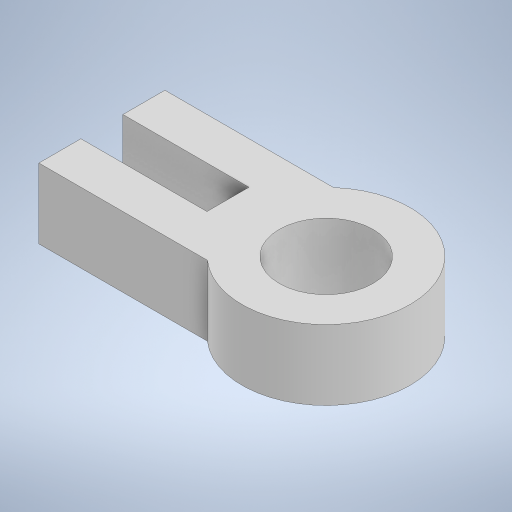
# Autodesk Inventor part: link_end_fixation
Saved by Autodesk Inventor 2024 (Build 280153000, 153)
## iProperties
Created: 2024-02-23
Part Number: link_end_fixation
Material: Generic
Document SubType Name: Modeling
Designer: clbri
Density: 1 g/cm^3
Appearance: Default
Author: clbri
Autodesk Inventor part; units mm, degrees
ref_plane "YZ Plane" through (0, 0, 0) normal (1, 0, 0) x (0, 1, 0)
ref_plane "XZ Plane" through (0, 0, 0) normal (0, 1, 0) x (-1, 0, 0)
ref_plane "XY Plane" through (0, 0, 0) normal (0, 0, 1) x (1, 0, 0)
sketch "Sketch1" plane through (0, 0, 0) normal (0, 0, 1) x (1, 0, 0)
  line L0 (0, 0) -> (13, 0)
  line L1 (13, 0) -> (13, 5)
  line L2 (13, 5) -> (0, 5)
  line L3 (0, 5) -> (0, 0)
  dimension "d0" = 13
  dimension "d1" = 5
  constraints: 8 end point, 2 parallel, 1 horizontal, 1 perpendicular
  measures "d0" distance of L2.end L1.end
  measures "d1" distance of L1.end L0.end
extrude "Extrusion1" add sketch "Sketch1" along normal blind 9
sketch "Sketch2" plane through (0, 5, 0) normal (0, 1, 0) x (1, 0, 0)
  line L0 (0, 0) -> (0, -9) projected
  line L1 (0, -6) -> (9, -6)
  line L2 (9, -6) -> (9, -3)
  line L3 (9, -3) -> (0, -3)
  line L4 (0, -3) -> (0, -6)
  line L5 (13, 0) -> (0, 0) projected
  point P0 (6.5, 0)
  point P1 (0, -3)
  dimension "d4" = 9
  dimension "d5" = 3
  dimension "d6" = 3
  constraints: 8 end point, 2 parallel, 1 horizontal, 1 midpoint, 1 perpendicular, 1 point on line
  measures "d4" distance of L3.end L2.end
  measures "d5" distance of L2.end L1.end
  measures "d6" distance from line of point (6.5, 0) L3
extrude "Extrusion2" cut sketch "Sketch2" against normal through all
sketch "Sketch3" plane through (0, 5, 0) normal (0, 1, 0) x (1, 0, 0)
  circle A0 centre (16, -4.5) radius 3.25
  circle A1 centre (16, -4.5) radius 6
  line L0 (9, -3) -> (9, -6) projected
  line L1 (13, 0) -> (0, 0) projected
  dimension "d9" = 6.5
  dimension "d10" = 12
  dimension "d11" = 7
  dimension "d12" = 4.5
  constraints: 2 centre point, 1 coincident
  measures "d9" diameter of A0
  measures "d10" diameter of A1
  measures "d11" distance from line of L0 A1.centre
  measures "d12" distance from line of L1 A0.centre
extrude "Extrusion3" add sketch "Sketch3" against normal blind 5
sketch "Sketch4" plane through (0, 5, 3) normal (0, 1, 0) x (1, 0, 0)
  circle A0 centre (16.0298, -1.52) radius 3.35
  point P0 (0, 3)
  dimension "d15" = 6.7
  constraints: 1 centre point
  measures "d15" diameter of A0
extrude "Extrusion4" cut sketch "Sketch4" against normal blind 10
body "Solid1"
